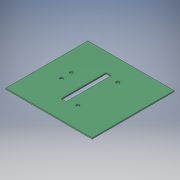
# Autodesk Inventor part: PCB
Saved by Autodesk Inventor 2017 (Build 210142000, 142)
## iProperties
Created: 2018-07-04
Part Number: PCB
Material: Generic
Document SubType Name: Modeling
Designer: intelsath
Density: 1 g/cm^3
Appearance: Default
Author: intelsath
Autodesk Inventor part; units mm, degrees
ref_plane "YZ Plane" through (0, 0, 0) normal (1, 0, 0) x (0, 1, 0)
ref_plane "XZ Plane" through (0, 0, 0) normal (0, 1, 0) x (-1, 0, 0)
ref_plane "XY Plane" through (0, 0, 0) normal (0, 0, 1) x (1, 0, 0)
sketch "Sketch1" plane through (0, 0, 0) normal (0, 1, 0) x (-1, 0, 0)
  line L0 (0, 0) -> (0, -54.66)
  line L1 (0, -54.66) -> (57.5, -54.66)
  line L2 (57.5, 0) -> (0, 0)
  line L3 (29.6, -12.35) -> (32.9, -12.35)
  line L4 (32.9, -12.35) -> (32.9, -42.35)
  line L5 (32.9, -42.35) -> (29.6, -42.35)
  line L6 (29.6, -42.35) -> (29.6, -12.35)
  line L7 (57.5, -54.66) -> (57.5, 0)
  circle A0 centre (44.5, -24.08) radius 1
  circle A1 centre (44.5, -30.58) radius 1
  circle A2 centre (23.5, -40.66) radius 1
  circle A3 centre (23.5, -14) radius 1
  point P0 (57.5, -27.33)
  point P1 (0, -27.33)
  dimension "d0" = 54.66
  dimension "d1" = 57.5
  dimension "d6" = 12.35
  dimension "d7" = 29.6
  dimension "d8" = 3.3
  dimension "d9" = 30
  dimension "d59" = 3.25
  dimension "d60" = 3.25
  dimension "d62" = 2
  dimension "d63" = 13.33
  dimension "d64" = 13.33
  dimension "d65" = 23.5
  dimension "d66" = 44.5
  constraints: 16 end point, 4 centre point, 4 perpendicular, 3 equal radius, 2 horizontal, 2 midpoint, 2 vertical, 2 vertical alignment
  measures "d0" distance of L0.start L0.end
  measures "d1" distance of L0.end L1.end
  measures "d6" distance from line of L2 L3.start
  measures "d7" distance between parallel lines of L0 L6
  measures "d8" distance of L4.end L5.end
  measures "d9" distance of L3.end L4.end
  measures "d59" vertical distance of point (57.5, -27.33) A0.centre
  measures "d60" vertical distance of point (57.5, -27.33) A1.centre
  measures "d62" diameter of A0
  measures "d63" vertical distance of point (0, -27.33) A2.centre
  measures "d64" vertical distance of point (0, -27.33) A3.centre
  measures "d65" distance from line of L0 A2.centre
  measures "d66" distance from line of L0 A1.centre
extrude "Extrusion2" add sketch "Sketch1" along normal blind 0.8
ref_plane "Work Plane1" through (0, 0.8, -27.33) normal (0, 0, 1) x (1, 0, 0)
equation "\"d64\" = d63"
body "Solid2"
